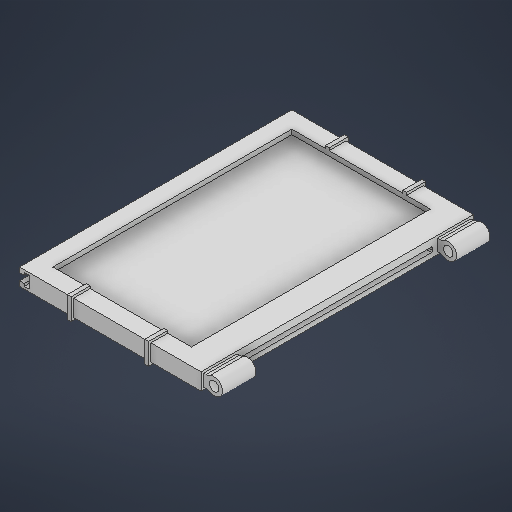
# Autodesk Inventor part: Дета2ль1
Saved by Autodesk Inventor 2025.1 (Build 291241000, 241)
## iProperties
Created: 2025-05-09
Part Number: Дета2ль1
Material: Типовые
Document SubType Name: Modeling
Designer: bogda
Density: 1 g/cm^3
Appearance: По умолчанию
Author: bogda
Autodesk Inventor part; units mm, degrees
ref_plane "YZ Plane" through (0, 0, 0) normal (1, 0, 0) x (0, 1, 0)
ref_plane "XZ Plane" through (0, 0, 0) normal (0, 1, 0) x (-1, 0, 0)
ref_plane "XY Plane" through (0, 0, 0) normal (0, 0, 1) x (1, 0, 0)
sketch "Эскиз1" plane through (0, 0, 0) normal (0, 1, 0) x (-1, 0, 0)
  line L0 (34, 53) -> (-34, 53)
  line L1 (-34, 53) -> (-34, -53)
  line L2 (-34, -53) -> (34, -53)
  line L3 (34, -53) -> (34, 53)
  line L4 (34, 53) -> (-34, -53) construction
  line L5 (-34, 53) -> (34, -53) construction
  line L6 (38, 57) -> (-38, 57)
  line L7 (-38, 57) -> (-38, -57)
  line L8 (-38, -57) -> (38, -57)
  line L9 (38, -57) -> (38, 57)
  point P0 (0, 0)
  dimension "d1" = 68
  dimension "d2" = 106
  dimension "d3" = 4
  constraints: 20 end point, 4 parallel, 2 midpoint, 2 perpendicular, 1 horizontal, 3 other
  measures "d1" distance of L2.end L1.end
  measures "d2" distance of L1.end L0.end
  measures "d3" distance between parallel lines of L3 L9
extrude "Выдавливание1" add sketch "Эскиз1" along normal blind 2 contours L3 L2 L1 L0
extrude "Выдавливание2" add sketch "Эскиз1" along normal blind 7
sketch "Эскиз2" plane through (0, 7, 0) normal (0, 1, 0) x (1, 0, 0)
  line L0 (34, -53) -> (-34, -53) projected
  line L1 (34, 53) -> (-34, 53)
  line L2 (-34, 53) -> (-34, -53)
  line L3 (-34, -53) -> (34, -53)
  line L4 (34, -53) -> (34, 53)
  line L5 (34, 53) -> (-34, -53) construction
  line L6 (-34, 53) -> (34, -53) construction
  line L7 (-34, -53) -> (-34, -50)
  line L8 (-34, -50) -> (34, -50)
  line L9 (-34, 53) -> (34, 53) projected
  line L10 (-34, 53) -> (-34, 50)
  line L11 (-34, 50) -> (34, 50)
  line L12 (34, 53) -> (34, -53) projected
  line L13 (34, -50) -> (27, -50)
  line L14 (27, -50) -> (27, 50)
  line L15 (-34, 50) -> (-31, 50)
  line L16 (-31, 50) -> (-31, -50)
  point P0 (0, 0)
  dimension "d8" = 3
  dimension "d9" = 3
  dimension "d10" = 7
  dimension "d11" = 3
  constraints: 28 end point, 8 point on line, 5 perpendicular, 2 midpoint, 2 parallel, 1 horizontal
  measures "d8" distance of L0.end L7.end
  measures "d9" distance of L1.end L10.end
  measures "d10" distance of L8.end L13.end
  measures "d11" distance of L10.end L15.end
extrude "Выдавливание3" add sketch "Эскиз2" against normal blind 2 contours L0 L2 L8 L4 | L8 L14 L11 L4 | L2 L11 L16 L8 | L11 L2 L1 L4
sketch "Эскиз3" plane through (38, 0, 57) normal (1, 0, 0) x (0, 0, -1)
  line L0 (114, 0) -> (0, 0) projected
  line L1 (0, 0) -> (16, 0)
  line L2 (16, 0) -> (16, 7)
  line L3 (114, 7) -> (0, 7) projected
  line L4 (114, 0) -> (114, 7) projected
  line L5 (114, 0) -> (98, 0)
  line L6 (98, 0) -> (98, 7)
  line L7 (98, 7) -> (114, 7)
  line L8 (114, 7) -> (114, 0)
  line L9 (0, 0) -> (0, 7)
  line L10 (0, 7) -> (16, 7)
  line L11 (15, 6) -> (15, 1)
  line L12 (15, 1) -> (1, 1)
  line L13 (1, 1) -> (1, 6)
  line L14 (1, 6) -> (15, 6)
  line L15 (99, 6) -> (99, 1)
  line L16 (99, 1) -> (113, 1)
  line L17 (113, 1) -> (113, 6)
  line L18 (113, 6) -> (99, 6)
  line L19 (16, 0) -> (17, 0)
  line L20 (17, 0) -> (17, 2)
  line L21 (98, 0) -> (97, 0)
  line L22 (97, 0) -> (97, 2)
  line L23 (96.5, 2) -> (17.5, 2)
  line L24 (17, 2.5) -> (17, 3.5)
  line L25 (17.5, 4) -> (96.5, 4)
  line L26 (97, 3.5) -> (97, 2.5)
  line L27 (110, 2) -> (4, 2) projected
  arc A0 (17.5, 4) -> (17, 3.5) centre (17.5, 3.5) ccw
  arc A1 (17, 2.5) -> (17.5, 2) centre (17.5, 2.5) ccw
  arc A2 (97, 3.5) -> (96.5, 4) centre (96.5, 3.5) ccw
  arc A3 (96.5, 2) -> (97, 2.5) centre (96.5, 2.5) ccw
  point P0 (57, 0)
  point P1 (17, 4)
  dimension "d14" = 16
  dimension "d15" = 16
  dimension "d16" = 1
  dimension "d17" = 1
  dimension "d18" = 1
  dimension "d19" = 2
  dimension "d20" = 1
  dimension "d21" = 2
  dimension "d22" = 2
  dimension "d23" = 0.5
  constraints: 48 end point, 13 perpendicular, 12 point on line, 8 point on circle, 8 tangent, 4 centre point, 3 equal radius, 3 parallel, 6 other
  measures "d14" distance of L0.end L1.end
  measures "d15" distance of L0.start L5.end
  measures "d16" distance between parallel lines of L2 L11
  measures "d17" distance between parallel lines of L6 L15
  measures "d18" distance of L1.end L19.end
  measures "d19" distance of L19.end L20.end
  measures "d20" distance of L5.end L21.end
  measures "d21" distance of L21.end L22.end
  measures "d22" distance of L20.end point (17, 4)
  measures "d23" radius of A0
extrude "Выдавливание4" cut sketch "Эскиз3" against normal blind 3 contours L23 A1 L24 A0 L25 A2 L26 A3
extrude "Выдавливание5" add sketch "Эскиз3" along normal blind 1 contours L15 L18 L17 L16 | L11 L12 L13 L14
sketch "Эскиз4" plane through (38, 0, -57) normal (0, 0, -1) x (-1, 0, 0)
  line L0 (0, 0) -> (76, 0) projected
  line L1 (76, 0) -> (76, 2)
  line L2 (76, 0) -> (76, 7) projected
  line L3 (72, 2) -> (72, 5) projected
  line L4 (76, 2) -> (72, 2)
  line L5 (72, 2) -> (72, 5)
  line L6 (72, 5) -> (76, 5)
  line L7 (76, 5) -> (76, 2)
  line L8 (72, 5) -> (72, 6)
  line L9 (72, 6) -> (74, 6)
  line L10 (74, 6) -> (74, 5)
  line L11 (74, 2) -> (74, 1)
  line L12 (74, 1) -> (72, 1)
  line L13 (72, 1) -> (72, 2)
  point P0 (38, 0)
  dimension "d28" = 2
  dimension "d29" = 1
  dimension "d30" = 2
  dimension "d31" = 1
  constraints: 22 end point, 5 point on line, 4 perpendicular, 2 midpoint
  measures "d28" distance of L0.end L1.end
  measures "d29" distance of L3.end L8.end
  measures "d30" distance of L8.end L9.end
  measures "d31" distance of L11.start L11.end
extrude "Выдавливание6" cut sketch "Эскиз4" against normal blind 120
sketch "Эскиз5" plane through (38, 1, 56) normal (0, 0, 1) x (1, 0, 0)
  line L0 (1, 5) -> (1, 0) projected
  line L1 (1, 0) -> (1, 2.5)
  line L2 (1, 2.5) -> (4.5, 2.5)
  circle A0 centre (4.5, 2.5) radius 3.5
  arc A1 (2.75, -0.5311) -> (1, 0) centre (0.4167, -5.0709) ccw
  arc A2 (1, 5) -> (2.6628, 5.479) centre (0.4389, 10.0731) ccw
  circle A3 centre (4.5, 2.5) radius 2
  point P0 (-38, -1)
  dimension "d34" = 2.5
  dimension "d36" = 3.5
  dimension "d37" = 5.104
  dimension "d38" = 4
  constraints: 6 point on circle, 4 centre point, 4 end point, 2 coincident, 1 horizontal, 1 midpoint
  measures "d34" distance of L0.end L1.end
  measures "d36" distance of L1.end L2.end
  measures "d37" radius of A2
  measures "d38" diameter of A3
extrude "Выдавливание7" add sketch "Эскиз5" against normal blind 112
sketch "Эскиз6" plane through (38, 1, 42) normal (0, 0, -1) x (-1, 0, 0)
  line L0 (0, 5) -> (-1, 5) projected
  line L1 (-1, 5) -> (-1, 8.1758)
  line L2 (-1, 8.1758) -> (-10.78, 8.3268)
  line L3 (-10.78, 8.3268) -> (-10.1005, -3.8271)
  line L4 (-10.1005, -3.8271) -> (-1.8469, -2.418)
  line L5 (-1.8469, -2.418) -> (-1, -0.011)
  line L6 (-1, -0.011) -> (-1, 5)
  point P0 (38, -1)
  constraints: 12 end point, 1 collinear, 1 point on line, 1 vertical
extrude "Выдавливание8" cut sketch "Эскиз6" along normal blind 84
sketch "Эскиз7" plane through (0, 0, 0) normal (0, -1, 0) x (1, 0, 0)
  circle A0 centre (0, 0) radius 34
  circle A1 centre (0, 0) radius 32.5
  line L0 (-17, -57.0311) -> (17, -57.0311)
  line L1 (-17, -57.0311) -> (-17, -35.0999)
  line L2 (-38, 57) -> (38, 57) projected
  line L3 (17, 57) -> (-17, 57)
  arc A2 (17, 35.0999) -> (-17, 35.0999) centre (0, 0) ccw
  arc A3 (-17, -35.0999) -> (17, -35.0999) centre (0, 0) ccw
  line L4 (-17, 35.0999) -> (-17, 57)
  line L5 (17, 35.0999) -> (17, 57)
  line L6 (17, -57.0311) -> (17, -35.0999)
  line L7 (-15.4, -37.5659) -> (-15.4, -55.4311)
  line L8 (15.4, -55.4311) -> (15.4, -37.5659)
  arc A4 (-15.4, -37.5659) -> (15.4, -37.5659) centre (0, 0) ccw
  line L9 (15.4, 55.4) -> (15.4, 37.5659)
  arc A5 (15.4, 37.5659) -> (-15.4, 37.5659) centre (0, 0) ccw
  line L10 (-15.4, 37.5659) -> (-15.4, 55.4)
  line L11 (-15.4, -55.4311) -> (-15.4, -57.0311)
  line L12 (15.4, -55.4311) -> (15.4, -57.0311)
  line L13 (-15.4, 55.4) -> (-15.4, 57)
  line L14 (15.4, 55.4) -> (15.4, 57)
  dimension "d43" = 65
  dimension "d51" = 1.6
  dimension "d52" = 1.6
  constraints: 28 end point, 8 point on circle, 8 point on line, 6 centre point, 3 perpendicular, 2 coincident, 2 vertical, 1 collinear, 3 other
  measures "d43" diameter of A1
  measures "d51" distance between parallel lines of L1 L7
  measures "d52" distance between parallel lines of L4 L10
extrude "Выдавливание9" add sketch "Эскиз7" along normal blind 1 contours A0 | L1 A3 L6 L0 L12 L8 A4 L7 L11 | L2 L13 L10 A5 L9 L14 L5 A2 L4
sketch "Эскиз8" plane through (-38, 7, 57) normal (0, 0, 1) x (1, 0, 0)
  line L0 (21, -7) -> (21, -8) projected
  line L1 (21, -8) -> (21, 0)
  line L2 (76, 0) -> (0, 0) projected
  line L3 (55, -8) -> (21, -8) projected
  line L4 (21, -8) -> (22.6, -8)
  line L5 (22.6, -8) -> (22.6, 0)
  line L6 (22.6, 0) -> (21, 0)
  line L7 (53.4, -7) -> (53.4, -8) projected
  line L8 (53.4, -8) -> (53.4, 0)
  line L9 (53.4, 0) -> (55, 0)
  line L10 (55, 0) -> (55, -8)
  line L11 (55, -8) -> (53.4, -8)
  point P0 (38, -7)
  dimension "d55" = 1.6
  dimension "d56" = 1.6
  constraints: 16 end point, 5 point on line, 4 perpendicular, 1 collinear, 1 vertical
  measures "d55" distance of L0.end L4.end
  measures "d56" distance of L8.end L9.end
extrude "Выдавливание10" add sketch "Эскиз8" along normal blind 1 contours L1 L2 L5 L3 L0 | L7 L8 L2 L10 L3
sketch "Эскиз9" plane through (38, 7, -57) normal (0, 0, -1) x (-1, 0, 0)
  line L0 (55, -7) -> (55, -8) projected
  line L1 (55, -8) -> (55, 0)
  line L2 (55, 0) -> (53.4, 0)
  line L3 (53.4, -7) -> (53.4, -8) projected
  line L4 (53.4, 0) -> (53.4, -8)
  line L5 (53.4, -8) -> (55, -8)
  line L6 (22.6, -7) -> (22.6, -8) projected
  line L7 (22.6, -8) -> (22.6, 0)
  line L8 (22.6, 0) -> (21, 0)
  line L9 (21, 0) -> (21, -8)
  line L10 (21, -8) -> (22.6, -8)
  point P0 (38, -7)
  dimension "d59" = 8
  dimension "d60" = 1.6
  dimension "d61" = 1.6
  constraints: 16 end point, 3 perpendicular, 3 point on line, 2 collinear
  measures "d59" distance of L0.end L1.end
  measures "d60" distance of L1.end L2.end
  measures "d61" distance of L7.end L8.end
extrude "Выдавливание11" add sketch "Эскиз9" along normal blind 1
sketch "Эскиз10" plane through (0, 7, 0) normal (0, 1, 0) x (1, 0, 0)
  line L0 (-15.4, -58) -> (-17, -58) projected
  line L1 (-17, -58) -> (-17, -50)
  line L2 (27, -50) -> (-31, -50) projected
  line L3 (-15.4, -57) -> (-15.4, -58) projected
  line L4 (-15.4, -58) -> (-17, -58)
  line L5 (-15.4, -58) -> (-15.4, -50)
  line L6 (-15.4, -50) -> (-17, -50)
  line L7 (15.4, -58) -> (15.4, -50)
  line L8 (15.4, -50) -> (17, -50)
  line L9 (17, -35.0999) -> (17, -58) projected
  line L10 (17, -58) -> (15.4, -58)
  line L11 (17, -58) -> (17, -50)
  line L12 (-17, 58) -> (-15.4, 58) projected
  line L13 (-17, 58) -> (-17, 50)
  line L14 (-17, 50) -> (-15.4, 50)
  line L15 (-15.4, 50) -> (-15.4, 58)
  line L16 (-15.4, 58) -> (-17, 58)
  line L17 (15.4, 58) -> (15.4, 50)
  line L18 (15.4, 50) -> (17, 50)
  line L19 (17, 58) -> (17, 50)
  line L20 (15.4, 58) -> (17, 58)
  point P0 (0, 0)
  dimension "d64" = 8
  constraints: 32 end point, 14 point on line, 7 perpendicular, 2 collinear, 2 vertical, 1 parallel
  measures "d64" distance of L17.start L17.end
extrude "Выдавливание12" add sketch "Эскиз10" along normal blind 1
